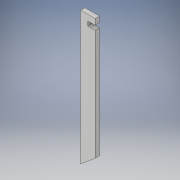
# Autodesk Inventor part: k2_t_leg
Saved by Autodesk Inventor 2017 (Build 210142000, 142)
## iProperties
Created: 2017-02-08
Part Number: k2_t_leg
Material: Generic
Document SubType Name: Modeling
Designer: herman
Density: 1 g/cm^3
Appearance: Default
Author: herman
Autodesk Inventor part; units mm, degrees
ref_plane "YZ Plane" through (0, 0, 0) normal (1, 0, 0) x (0, 1, 0)
ref_plane "XZ Plane" through (0, 0, 0) normal (0, 1, 0) x (-1, 0, 0)
ref_plane "XY Plane" through (0, 0, 0) normal (0, 0, 1) x (1, 0, 0)
sketch "Sketch2" plane through (0, 0, 0) normal (0, 0, 1) x (1, 0, 0)
  line L0 (-2.2295, 56.043) -> (-2.2295, -36.5452)
  line L1 (-2.2295, -36.5452) -> (7.7705, -28.1542)
  line L2 (7.7705, -28.1542) -> (7.7705, 49.043)
  line L3 (7.7705, 49.043) -> (2.7705, 49.043)
  line L4 (2.7705, 49.043) -> (2.7705, 52.043)
  line L5 (2.7705, 52.043) -> (7.7705, 52.043)
  line L6 (7.7705, 52.043) -> (7.7705, 56.043)
  line L7 (7.7705, 56.043) -> (-2.2295, 56.043)
  point P0 (0, 0)
  dimension "d1" = 5
  dimension "d2" = 3
  dimension "d3" = 130
  dimension "d4" = 4
  dimension "d5" = 5
  dimension "d6" = 77.1972
  constraints: 16 end point, 5 perpendicular, 4 point on line, 1 parallel, 1 vertical
  measures "d1" distance of L4.end L5.end
  measures "d2" distance of L3.end L4.end
  measures "d3" angle of L2 L1
  measures "d4" distance of L5.end L6.end
  measures "d5" horizontal distance of L4.end L0.start
  measures "d6" distance of L2.end L1.end
extrude "Extrusion1" add sketch "Sketch2" along normal blind 3
body "Solid2"
